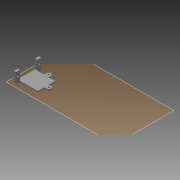
# Autodesk Inventor part: soporteIzq
Saved by Autodesk Inventor 2015 (Build 190159000, 159)
## iProperties
Created: 2015-02-22
Part Number: soporteIzq
Material: Genérico
Document SubType Name: Modeling
Designer: jorge
Density: 1 g/cm^3
Appearance: Valor por defecto
Author: jorge
Autodesk Inventor part; units mm, degrees
ref_plane "YZ Plane" through (0, 0, 0) normal (1, 0, 0) x (0, 1, 0)
ref_plane "XZ Plane" through (0, 0, 0) normal (0, 1, 0) x (-1, 0, 0)
ref_plane "XY Plane" through (0, 0, 0) normal (0, 0, 1) x (1, 0, 0)
sketch "Boceto2" plane through (0, 0, 0) normal (0, 0, 1) x (1, 0, 0)
  circle A0 centre (60.5, -11.7293) radius 1.25 projected
  circle A1 centre (60.5, -32) radius 1.25 projected
  line L0 (-63.5, 34.5) -> (63.5, 34.5) projected
  line L1 (-63.5, -34.5) -> (-63.5, 34.5) projected
  line L2 (63.5, -34.5) -> (-63.5, -34.5) projected
  line L3 (63.5, 34.5) -> (63.5, -34.5) projected
  line L4 (-37.2586, -7.2586) -> (-37.2586, -29.3586) projected
  line L5 (-58.4586, -34.5586) -> (-60.3586, -34.5586) projected
  line L6 (-70.2586, -17.8586) -> (-70.2586, -21.2586) projected
  line L7 (-60.3586, -2.2586) -> (-58.4586, -2.2586) projected
  line L8 (-58.4586, -2.2586) -> (-58.4586, -34.3586) projected
  line L9 (-60.3586, -34.3586) -> (-60.3586, -29.3586) projected
  line L10 (-60.5586, -2.2586) -> (-60.5586, -6.8586) projected
  line L11 (-60.5586, -2.2586) -> (-63.5, -2.2586)
  line L12 (-63.5, -2.2586) -> (-63.5, -34.5)
  line L13 (-63.5, -34.5) -> (-60.5586, -34.5)
  line L14 (-60.5586, -34.5) -> (-60.5586, -2.2586)
  circle A2 centre (-49.0086, -4.2586) radius 1 projected
  circle A3 centre (-34.4586, -18.4086) radius 1 projected
  point P0 (0, 0)
  constraints: 8 end point, 2 parallel, 1 horizontal, 1 perpendicular
ref_plane "Plano de trabajo1" through (-63.7586, -34.3586, 1.8) normal (0, 0, -1) x (0, 1, 0)
extrude "Extrusión1" add sketch "Boceto2" along normal up to surface (1.8 mm away) contours L11 L10 L14 L2 L1
sketch "Boceto3" plane through (-63.5, -34.5, 1.8) normal (0, 0, 1) x (1, 0, 0)
  line L0 (2.9414, 4.9414) -> (-0.2586, 4.9414) projected
  line L1 (-0.0586, 27.4414) -> (2.7414, 27.4414) projected
  line L2 (-0.0586, 27.4414) -> (2.9414, 27.4414)
  line L3 (2.9414, 27.4414) -> (2.9414, 32.2414)
  line L4 (2.9414, 32.2414) -> (-0.0586, 32.2414)
  line L5 (-0.0586, 32.2414) -> (-0.0586, 27.4414)
  line L6 (-0.2586, 4.9414) -> (2.9414, 4.9414)
  line L7 (2.9414, 4.9414) -> (2.9414, 0)
  line L8 (2.9414, 0) -> (-0.2586, 0)
  line L9 (-0.2586, 0) -> (-0.2586, 4.9414)
  point P0 (63.5, 34.5)
  constraints: 16 end point, 4 parallel, 2 horizontal, 2 perpendicular
ref_plane "Plano de trabajo2" through (-63.7586, -34.3586, 13.8) normal (0, 0, -1) x (0, 1, 0)
extrude "Extrusión2" add sketch "Boceto3" along normal up to surface (12 mm away)
sketch "Boceto4" plane through (-63.5586, -7.0586, 1.8) normal (-1, 0, 0) x (0, 0, 1)
  arc A0 (5.3, 3.7247) -> (6.7, 3.7247) centre (6, 2.75) ccw projected
  arc A1 (6.5, -26.3409) -> (5.3, -26.2247) centre (6, -25.25) ccw projected
  arc A2 (6.5, -26.3409) -> (5.3, -26.2247) centre (6, -25.25) ccw projected
  arc A3 (6.5, -26.3409) -> (5.3, -26.2247) centre (6, -25.25) ccw projected
  point P0 (-1.8, 7.0586)
hole "Agujero1" at (-63.5586, -4.3086, 7.8) direction (1, 0, 0) diameter 2 end up to face face through (-60.5586, -32.8529, 5.2) facing (1, 0, 0)
sketch "Boceto5" plane through (-63.7586, -34.5, 1.8) normal (-1, 0, 0) x (0, 0, 1)
  arc A0 (6.5, 1.1006) -> (5.3, 1.2167) centre (6, 2.1914) ccw projected
  point P0 (-1.8, 34.5)
hole "Agujero2" at (-63.7586, -32.3086, 7.8) direction (1, 0, 0) diameter 2 end up to face face through (-60.5586, -32.8529, 5.2) facing (1, 0, 0)
move faces "Desplazar1" translate (-0.0586, 0, 0) faces at (-63.5, -14.6057, 0.6)
move faces "Desplazar2" translate (0.2, 0, 0) faces at (-63.7586, -32.1224, 3.4667)
ref_plane "Plano de trabajo3" through (0, 0, 0) normal (0, 0, 1) x (1, 0, 0)
sketch "Boceto6" plane through (0, 0, 0) normal (0, 0, 1) x (1, 0, 0)
  line L0 (-37.4586, -7.2586) -> (-37.4586, -29.3586) projected
  line L1 (-37.4586, -29.3586) -> (-37.4586, -38.3484)
  circle A0 centre (60.5, -11.7293) radius 1.25 projected
  circle A1 centre (60.5, -32) radius 1.25 projected
  line L2 (-63.5, 34.5) -> (63.5, 34.5) projected
  line L3 (-63.5, -34.5) -> (-63.5, 34.5) projected
  line L4 (63.5, -34.5) -> (-63.5, -34.5) projected
  line L5 (63.5, 34.5) -> (63.5, -34.5) projected
  line L6 (-58.0586, -7.2586) -> (-37.4586, -7.2586) projected
  line L7 (-58.0586, -29.5586) -> (-37.4586, -29.5586) projected
  line L8 (-37.4586, -29.5586) -> (-60.5586, -29.5586)
  line L9 (-60.5586, -34.5) -> (-60.5586, -2.2586) projected
  line L10 (-60.5586, -29.5586) -> (-37.4586, -29.5586)
  line L11 (-37.4586, -29.5586) -> (-37.4586, -7.2586)
  line L12 (-37.4586, -7.2586) -> (-60.5586, -7.2586)
  line L13 (-60.5586, -7.2586) -> (-60.5586, -29.5586)
  circle A2 centre (-49.0086, -4.2586) radius 1 projected
  circle A3 centre (-34.4586, -18.4086) radius 1 projected
  point P0 (0, 0)
  constraints: 12 end point, 2 horizontal, 2 parallel, 1 perpendicular, 1 point on line, 1 vertical
ref_plane "Plano de trabajo4" through (-58.0586, -29.3586, 1.8) normal (0, 0, 1) x (1, 0, 0)
extrude "Extrusión3" add sketch "Boceto6" along normal up to surface (1.8 mm away) contours L0 L1 L7 L8 L9 L12 L6
sketch "Boceto7" plane through (-37.4586, -29.5586, 0) normal (1, 0, 0) x (0, 0, -1)
  line L0 (-1.8, 0) -> (-1.8, 22.3)
  line L1 (-1.8, 22.3) -> (-1.8, 0) projected
  line L2 (-1.8, 11.15) -> (0, 11.15)
  line L3 (0, 0) -> (0, 22.3) projected
  line L4 (0, 8.15) -> (-1.8, 8.15)
  line L5 (-1.8, 8.15) -> (-1.8, 14.15)
  line L6 (-1.8, 14.15) -> (0, 14.15)
  line L7 (0, 14.15) -> (0, 8.15)
  line L8 (0, 8.15) -> (-1.8, 14.15) construction
  line L9 (-1.8, 8.15) -> (0, 14.15) construction
  point P0 (0, 29.5586)
  point P1 (-0.9, 11.15)
  dimension "d26" = 6
  constraints: 16 end point, 5 midpoint, 3 equal length, 1 horizontal, 1 perpendicular, 1 point on line
  measures "d26" distance of L4.end L5.end
extrude "Extrusión4" add sketch "Boceto7" along normal blind 6
sketch "Boceto8" plane through (-63.5586, -7.0586, 1.8) normal (0, 0, 1) x (1, 0, 0)
  line L0 (26.1, -14.35) -> (26.1, -8.35)
  line L1 (26.1, -14.35) -> (29.1, -14.35)
  line L2 (26.1, -14.35) -> (32.1, -14.35) projected
  line L3 (26.1, -8.35) -> (32.1, -8.35) projected
  line L4 (29.1, -8.35) -> (29.1, -14.35)
  arc A0 (29.1, -14.35) -> (29.1, -8.35) centre (29.1, -11.35) ccw
  line L5 (32.1, -14.35) -> (32.1, -8.35)
  line L6 (29.1, -8.35) -> (32.0071, -8.35)
  line L7 (29.1, -14.35) -> (32.1, -14.35)
  point P0 (63.5586, 7.0586)
  constraints: 12 end point, 4 midpoint, 2 point on circle, 2 vertical, 1 centre point, 1 collinear, 1 perpendicular, 1 point on line, 1 tangent
ref_plane "Plano de trabajo5" through (-63.5, -34.5, 0) normal (0, 0, 1) x (1, 0, 0)
extrude "Extrusión5" cut sketch "Boceto8" against normal up to surface (1.8 mm away) contours A0 L5 L2 | L3 L5 A0
hole "Agujero3" at (-34.4586, -18.4086, 1.8) direction (0, 0, -1) diameter 2 depth 1.8 tip angle 118
sketch "Boceto10" plane through (-60.5586, -7.2586, 0) normal (0, 1, 0) x (1, 0, 0)
  line L0 (23.1, 0) -> (0, 0) projected
  line L1 (11.55, 0) -> (11.55, -1.8)
  line L2 (0, -1.8) -> (23.1, -1.8) projected
  line L3 (14.55, -1.8) -> (8.55, -1.8)
  line L4 (8.55, -1.8) -> (8.55, 0)
  line L5 (8.55, 0) -> (14.55, 0)
  line L6 (14.55, 0) -> (14.55, -1.8)
  line L7 (14.55, -1.8) -> (8.55, 0) construction
  line L8 (8.55, -1.8) -> (14.55, 0) construction
  point P0 (60.5586, 0)
  point P1 (11.55, -0.9)
  dimension "d40" = 6
  constraints: 14 end point, 5 midpoint, 2 parallel, 1 horizontal, 1 perpendicular, 1 point on line
  measures "d40" distance of L4.end L5.end
extrude "Extrusión6" add sketch "Boceto10" along normal blind 6
sketch "Boceto11" plane through (-63.5586, -7.0586, 1.8) normal (0, 0, 1) x (1, 0, 0)
  line L0 (17.55, -0.2) -> (17.55, 5.8) projected
  line L1 (17.55, 2.8) -> (11.55, 2.8)
  line L2 (11.55, -0.2) -> (11.55, 5.8) projected
  arc A0 (17.55, 2.8) -> (11.55, 2.8) centre (14.55, 2.8) ccw
  line L3 (17.55, 5.8) -> (11.55, 5.8)
  line L4 (11.55, 2.8) -> (11.55, 5.8)
  line L5 (11.55, 5.8) -> (17.55, 5.8) projected
  line L6 (17.55, 2.8) -> (17.55, 5.8)
  point P0 (63.5586, 7.0586)
  constraints: 8 end point, 3 midpoint, 2 point on circle, 1 centre point, 1 horizontal, 1 parallel, 1 perpendicular
ref_plane "Plano de trabajo6" through (-63.5, -34.5, 0) normal (0, 0, 1) x (1, 0, 0)
extrude "Extrusión7" cut sketch "Boceto11" against normal up to surface (1.8 mm away) contours A0 L3 L0 | L2 L3 A0
hole "Agujero4" at (-49.0086, -4.2586, 1.8) direction (0, 0, -1) diameter 2 depth 1.8 tip angle 118
